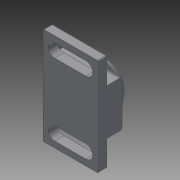
# Autodesk Inventor part: button
Saved by Autodesk Inventor 2015 SP1 (Build 190203100, 203)
## iProperties
Created: 2018-04-16
Part Number: button
Material: Generic
Document SubType Name: Modeling
Designer: 407642
Density: 1 g/cm^3
Appearance: Default
Author: 407642
Autodesk Inventor part; units mm, degrees
ref_plane "YZ Plane" through (0, 0, 0) normal (1, 0, 0) x (0, 1, 0)
ref_plane "XZ Plane" through (0, 0, 0) normal (0, 1, 0) x (-1, 0, 0)
sketch "Sketch1" plane through (0, 0, 0) normal (0, 1, 0) x (-1, 0, 0)
  line L0 (0, 0) -> (30, 0)
  line L1 (30, 0) -> (30, -53)
  line L2 (30, -53) -> (0, -53)
  line L3 (0, -53) -> (0, 0)
  dimension "d0" = 30
  dimension "d1" = 53
  constraints: 8 end point, 2 parallel, 1 horizontal, 1 perpendicular
  measures "d0" distance of L1.end L2.end
  measures "d1" distance of L0.end L1.end
extrude "Extrusion1" add sketch "Sketch1" along normal blind 5
sketch "Sketch2" plane through (0, 5, 0) normal (0, 1, 0) x (1, 0, 0)
  line L0 (-30, 53) -> (-30, 0) projected
  line L1 (0, 53) -> (-30, 53)
  line L2 (-30, 53) -> (-30, 39)
  line L3 (-30, 39) -> (0, 39)
  line L4 (0, 39) -> (0, 53)
  line L5 (0, 0) -> (-30, 0)
  line L6 (-30, 0) -> (-30, 14)
  line L7 (-30, 14) -> (0, 14)
  line L8 (0, 14) -> (0, 0)
  line L9 (0, 39) -> (-30, 39)
  line L10 (-30, 39) -> (-30, 14)
  line L11 (-30, 14) -> (0, 14)
  line L12 (0, 14) -> (0, 39)
  dimension "d4" = 14
  dimension "d5" = 14
  constraints: 24 end point, 6 parallel, 3 horizontal, 3 perpendicular, 2 point on line
  measures "d4" distance of L2.end L1.end
  measures "d5" distance of L5.end L6.end
extrude "Extrusion2" add sketch "Sketch2" along normal blind 8 contours L3 L12 L7 L0
sketch "Sketch3" plane through (0, 13, 0) normal (0, 1, 0) x (1, 0, 0)
  circle A0 centre (-15, 26.5) radius 7.5
  point P0 (0, 0)
  dimension "d8" = 15
  constraints: 1 centre point
  measures "d8" diameter of A0
extrude "Extrusion3" add sketch "Sketch3" along normal blind 3
ref_plane "Work Plane1" through (-15, 0, -53) normal (-1, 0, 0) x (0, 0, 1)
sketch "Sketch4" plane through (-15, 0, -53) normal (-1, 0, 0) x (0, 0, 1)
  line L0 (19, 16) -> (26.5, 16)
  line L1 (14, 5) -> (14, 13) projected
  line L2 (39, 5) -> (39, 13) projected
  line L3 (53, 0) -> (0, 0) projected
  line L4 (53, 0) -> (53, 5) projected
  line L5 (39, 5) -> (53, 5) projected
  line L6 (39, 5) -> (39, 13) projected
  line L7 (14, 13) -> (39, 13) projected
  line L8 (14, 5) -> (14, 13) projected
  line L9 (0, 5) -> (14, 5) projected
  line L10 (0, 0) -> (0, 5) projected
  line L11 (26.5, 16) -> (14, 16)
  line L12 (26.5, 16) -> (26.5, 21)
  arc A0 (21.1584, 21) -> (14, 16) centre (20.9681, 13.6482) ccw
  line L13 (21.1584, 21) -> (26.5, 21)
  constraints: 8 end point, 3 horizontal, 2 point on circle, 1 centre point, 1 vertical
revolve "Revolution1" add sketch "Sketch4" angle 360 about axis through (-15, 16, -26.5) along (0, 1, 0) contours L11 A0 L13 L12 L0
sketch "Sketch5" plane through (0, 5, 0) normal (0, 1, 0) x (1, 0, 0)
  line L0 (-6.6727, 10.5436) -> (-23.7046, 10.5436)
  line L1 (-23.7046, 3.3179) -> (-6.6727, 3.3179)
  arc A0 (-6.6727, 3.3179) -> (-6.6727, 10.5436) centre (-6.6727, 6.9307) ccw
  arc A1 (-23.7046, 10.5436) -> (-23.7046, 3.3179) centre (-23.7046, 6.9307) ccw
  line L2 (0, 14) -> (0, 39) projected
  line L3 (0, 26.5) -> (-37.5908, 26.5)
  line L4 (-6.6727, 42.4564) -> (-23.7046, 42.4564)
  line L5 (-23.7046, 49.6821) -> (-6.6727, 49.6821)
  arc A2 (-6.6727, 42.4564) -> (-6.6727, 49.6821) centre (-6.6727, 46.0693) ccw
  arc A3 (-23.7046, 49.6821) -> (-23.7046, 42.4564) centre (-23.7046, 46.0693) ccw
  point P0 (0, 0)
  constraints: 10 end point, 8 point on circle, 6 symmetric about line, 4 centre point, 4 tangent, 2 horizontal, 1 midpoint, 1 parallel, 2 other
extrude "Extrusion4" cut sketch "Sketch5" against normal blind 32
fillet "Fillet1" radius 0.5 10 edges at (0, 5, -7) (-30, 5, -7) (-15, 5, 0) (0, 5, -46) (-15, 5, -53) (-30, 5, -46) (-30, 2.5, -53) (-30, 2.5, 0) (0, 2.5, 0) (0, 2.5, -53)
fillet "Fillet2" radius 1.5 2 edges at (-15, 13, -14) (-15, 13, -39)
body "Solid1"
